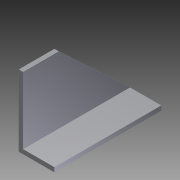
# Autodesk Inventor part: manipulator corner brace right
Saved by Autodesk Inventor 2012 (Build 160160000, 160)
## iProperties
Created: 2013-10-02
Part Number: manipulator corner brace right
Material: Default
Document SubType Name: Modeling
Designer: Bryce
Density: 1 g/cm^3
Author: Bryce
Autodesk Inventor part; units mm, degrees
ref_plane "YZ Plane" through (0, 0, 0) normal (1, 0, 0) x (0, 1, 0)
ref_plane "XZ Plane" through (0, 0, 0) normal (0, 1, 0) x (-1, 0, 0)
ref_plane "XY Plane" through (0, 0, 0) normal (0, 0, 1) x (1, 0, 0)
sketch "Sketch1" plane through (0, 0, 0) normal (0, 0, 1) x (1, 0, 0)
  line L0 (0, 0) -> (25.4, 0)
  line L1 (25.4, 0) -> (25.4, 3.1546)
  line L2 (3.1546, 50.8) -> (0, 50.8)
  line L3 (0, 50.8) -> (0, 0)
  line L4 (3.1546, 50.8) -> (3.1546, 3.1546)
  line L5 (3.1546, 3.1546) -> (25.4, 3.1546)
  dimension "d0" = 50.8
  dimension "d1" = 25.4
  dimension "d2" = 3.1546
  constraints: 12 end point, 4 parallel, 2 perpendicular, 1 horizontal
  measures "d0" distance of L2.end L0.start
  measures "d1" distance of L0.start L0.end
  measures "d2" distance of L2.start L2.end
extrude "Extrusion1" add sketch "Sketch1" along normal blind 76.2
sketch "Sketch2" plane through (0, 0, 0) normal (-1, 0, 0) x (0, 0, 1)
  line L0 (76.2, 0) -> (76.2, 50.8) projected
  line L1 (0, 50.8) -> (76.2, 50.8) projected
  line L2 (0, 50.8) -> (0, 0) projected
  line L3 (0, 0) -> (76.2, 0) projected
  line L4 (50.8, 50.8) -> (50.8, 0) construction
  line L5 (50.8, 50.8) -> (0, 3.175)
  dimension "d5" = 25.4
  dimension "d6" = 3.175
  constraints: 4 end point, 3 point on line, 1 perpendicular
  measures "d5" distance between parallel lines of L0 L4
  measures "d6" distance of L2.end L5.end
extrude "Extrusion2" cut sketch "Sketch2" against normal blind 25.4 contours L5 L2 L1
body "Solid1"
